Autodesk Inventor part; units mm, degrees
(part 3 of 3)
  spline S597 degree 2 poles (111.3325, 10.8139) (111.3763, 10.2474) (111.3763, 9.9326) knots 0 0 0 1 1 1
  spline S598 degree 2 poles (111.3763, 9.9326) (111.3763, 9.8642) (111.4037, 9.585) (111.4037, 9.5138) knots 0 0 0 1 2 2 2
  spline S599 degree 2 poles (111.4037, 9.5138) (111.4037, 9.3824) (111.3599, 9.2839) knots 0 0 0 1 1 1
  spline S600 degree 2 poles (111.3599, 9.2839) (111.3052, 9.1553) (111.1902, 9.1553) knots 0 0 0 1 1 1
  spline S601 degree 2 poles (111.1902, 9.1553) (111.1108, 9.1553) (110.9849, 9.2648) (110.9849, 9.3523) knots 0 0 0 1 2 2 2
  spline S602 degree 2 poles (110.9849, 9.3523) (110.9849, 9.3824) (111.0041, 9.5001) (111.0041, 9.5275) knots 0 0 0 1 2 2 2
  spline S603 degree 2 poles (111.0041, 9.5275) (111.0041, 9.626) (110.9794, 10.0092) (110.9794, 10.1078) knots 0 0 0 1 2 2 2
  spline S604 degree 2 poles (110.9794, 10.1078) (110.9794, 10.3897) (110.9329, 10.8988) knots 0 0 0 1 1 1
  spline S605 degree 2 poles (110.9329, 10.8988) (110.8864, 11.4462) (110.8809, 11.6871) knots 0 0 0 1 1 1
  line L469 (110.8809, 11.6871) -> (110.703, 11.6843)
  spline S606 degree 2 poles (110.703, 11.6843) (110.2733, 11.6843) (110.0269, 11.7473) knots 0 0 0 1 1 1
  spline S607 degree 2 poles (110.0269, 11.7473) (109.8682, 11.7883) (109.8682, 11.9416) knots 0 0 0 1 1 1
  spline S608 degree 2 poles (109.8682, 11.9416) (109.8682, 12.0237) (109.9202, 12.0839) knots 0 0 0 1 1 1
  spline S609 degree 2 poles (109.9202, 12.0839) (109.9777, 12.1524) (110.0707, 12.1469) knots 0 0 0 1 1 1
  spline S610 degree 2 poles (110.0707, 12.1469) (110.1392, 12.1441) (110.3855, 12.1113) knots 0 0 0 1 1 1
  spline S611 degree 2 poles (110.3855, 12.1113) (110.5798, 12.0867) (110.703, 12.0867) knots 0 0 0 1 1 1
  spline S612 degree 2 poles (110.703, 12.0867) (110.8207, 12.0867) (111.2997, 12.0976) (111.4174, 12.0976) knots 0 0 0 1 2 2 2
  spline S613 degree 2 poles (111.4174, 12.0976) (111.5679, 12.0976) (112.1619, 12.0538) (112.3151, 12.0538) knots 0 0 0 1 2 2 2
  spline S614 degree 2 poles (112.3151, 12.0538) (112.3972, 12.0538) (112.5122, 11.9389) (112.5122, 11.8513) knots 0 0 0 1 2 2 2
  spline S615 degree 2 poles (112.5122, 11.8513) (112.5122, 11.7692) (112.3972, 11.6515) (112.3151, 11.6515) knots 0 0 0 1 2 2 2
  spline S616 degree 2 poles (113.9464, 9.0513) (113.3935, 9.0513) (113.0076, 9.3824) knots 0 0 0 1 1 1
  spline S617 degree 2 poles (113.0076, 9.3824) (112.5998, 9.7355) (112.5998, 10.2939) knots 0 0 0 1 1 1
  spline S618 degree 2 poles (112.5998, 10.2939) (112.5998, 10.9754) (113.0021, 11.531) knots 0 0 0 1 1 1
  spline S619 degree 2 poles (113.0021, 11.531) (113.451, 12.1469) (114.1243, 12.1469) knots 0 0 0 1 1 1
  spline S620 degree 2 poles (114.1243, 12.1469) (114.7675, 12.1469) (115.0823, 11.8568) knots 0 0 0 1 1 1
  spline S621 degree 2 poles (115.0823, 11.8568) (115.4108, 11.5529) (115.4108, 10.9015) knots 0 0 0 1 1 1
  spline S622 degree 2 poles (115.4108, 10.9015) (115.4108, 10.2227) (115.0412, 9.6753) knots 0 0 0 1 1 1
  spline S623 degree 2 poles (115.0412, 9.6753) (114.617, 9.0513) (113.9464, 9.0513) knots 0 0 0 1 1 1
  spline S624 degree 2 poles (114.1243, 11.7445) (113.6426, 11.7445) (113.3087, 11.2655) knots 0 0 0 1 1 1
  spline S625 degree 2 poles (113.3087, 11.2655) (112.9994, 10.8249) (112.9994, 10.2939) knots 0 0 0 1 1 1
  spline S626 degree 2 poles (112.9994, 10.2939) (112.9994, 9.9162) (113.2813, 9.678) knots 0 0 0 1 1 1
  spline S627 degree 2 poles (113.2813, 9.678) (113.5495, 9.4536) (113.9464, 9.4536) knots 0 0 0 1 1 1
  spline S628 degree 2 poles (113.9464, 9.4536) (114.4227, 9.4536) (114.7347, 9.9353) knots 0 0 0 1 1 1
  spline S629 degree 2 poles (114.7347, 9.9353) (115.0111, 10.3651) (115.0111, 10.9015) knots 0 0 0 1 1 1
  spline S630 degree 2 poles (115.0111, 10.9015) (115.0111, 11.3723) (114.8004, 11.5612) knots 0 0 0 1 1 1
  spline S631 degree 2 poles (114.8004, 11.5612) (114.6006, 11.7445) (114.1243, 11.7445) knots 0 0 0 1 1 1
  spline S632 degree 2 poles (102.0155, 2.4094) (101.9416, 2.4094) (101.8759, 2.4724) knots 0 0 0 1 1 1
  spline S633 degree 2 poles (101.8759, 2.4724) (101.2273, 3.1128) (100.4308, 3.3345) knots 0 0 0 1 1 1
  line L470 (100.4308, 3.3345) -> (100.4472, 2.9513)
  line L471 (100.4472, 2.9513) -> (100.4581, 2.5654)
  spline S634 degree 2 poles (100.4581, 2.5654) (100.4581, 2.4778) (100.3459, 2.3629) (100.2611, 2.3629) knots 0 0 0 1 2 2 2
  spline S635 degree 2 poles (100.2611, 2.3629) (100.1762, 2.3629) (100.064, 2.4778) (100.064, 2.5654) knots 0 0 0 1 2 2 2
  spline S636 degree 2 poles (100.064, 2.5654) (100.064, 2.7214) (100.0339, 3.3345) (100.0339, 3.4905) knots 0 0 0 1 2 2 2
  spline S637 degree 2 poles (100.0339, 3.4905) (100.0339, 3.6712) (100.1133, 4.3856) (100.1133, 4.5635) knots 0 0 0 1 2 2 2
  spline S638 degree 2 poles (100.1133, 4.5635) (100.1133, 4.6647) (100.075, 5.0561) (100.075, 5.1574) knots 0 0 0 1 2 2 2
  spline S639 degree 2 poles (100.075, 5.1574) (100.075, 5.2696) (100.1379, 5.3545) knots 0 0 0 1 1 1
  spline S640 degree 2 poles (100.1379, 5.3545) (100.2118, 5.4585) (100.3432, 5.4475) knots 0 0 0 1 1 1
  line L472 (100.3432, 5.4475) -> (100.8167, 5.4092)
  spline S641 degree 2 poles (100.8167, 5.4092) (101.0849, 5.3764) (101.2711, 5.2778) knots 0 0 0 1 1 1
  spline S642 degree 2 poles (101.2711, 5.2778) (102.0648, 4.8563) (102.0648, 4.2487) knots 0 0 0 1 1 1
  spline S643 degree 2 poles (102.0648, 4.2487) (102.0648, 3.9504) (101.7938, 3.7205) knots 0 0 0 1 1 1
  spline S644 degree 2 poles (101.7938, 3.7205) (101.5776, 3.5343) (101.2519, 3.4385) knots 0 0 0 1 1 1
  spline S645 degree 2 poles (101.2519, 3.4385) (101.8623, 3.1101) (102.1633, 2.7461) knots 0 0 0 1 1 1
  spline S646 degree 2 poles (102.1633, 2.7461) (102.2153, 2.6831) (102.2153, 2.6147) knots 0 0 0 1 1 1
  spline S647 degree 2 poles (102.2153, 2.6147) (102.2153, 2.5298) (102.0949, 2.4094) (102.0155, 2.4094) knots 0 0 0 1 2 2 2
  line L473 (100.7647, 5.0041) -> (100.4746, 5.0288)
  line L474 (100.4746, 5.0288) -> (100.4937, 4.7907)
  spline S648 degree 2 poles (100.4937, 4.7907) (100.5074, 4.6456) (100.5074, 4.5525) knots 0 0 0 1 1 1
  spline S649 degree 2 poles (100.5074, 4.5525) (100.5074, 4.3965) (100.4828, 4.1611) knots 0 0 0 1 1 1
  line L475 (100.4828, 4.1611) -> (100.4417, 3.7697)
  spline S650 degree 2 poles (100.4417, 3.7697) (100.4691, 3.7697) (100.5841, 3.767) (100.6142, 3.767) knots 0 0 0 1 2 2 2
  spline S651 degree 2 poles (100.6142, 3.767) (101.115, 3.767) (101.3641, 3.9011) knots 0 0 0 1 1 1
  spline S652 degree 2 poles (101.3641, 3.9011) (101.4736, 3.9613) (101.5667, 4.0599) knots 0 0 0 1 1 1
  spline S653 degree 2 poles (101.5667, 4.0599) (101.6707, 4.1693) (101.6707, 4.246) knots 0 0 0 1 1 1
  spline S654 degree 2 poles (101.6707, 4.246) (101.6707, 4.5197) (101.3614, 4.7551) knots 0 0 0 1 1 1
  spline S655 degree 2 poles (101.3614, 4.7551) (101.0767, 4.9713) (100.7647, 5.0041) knots 0 0 0 1 1 1
  spline S656 degree 2 poles (103.9041, 2.3109) (103.3512, 2.3109) (102.9653, 2.6421) knots 0 0 0 1 1 1
  spline S657 degree 2 poles (102.9653, 2.6421) (102.5575, 2.9951) (102.5575, 3.5535) knots 0 0 0 1 1 1
  spline S658 degree 2 poles (102.5575, 3.5535) (102.5575, 4.235) (102.9598, 4.7907) knots 0 0 0 1 1 1
  spline S659 degree 2 poles (102.9598, 4.7907) (103.4087, 5.4065) (104.082, 5.4065) knots 0 0 0 1 1 1
  spline S660 degree 2 poles (104.082, 5.4065) (104.7252, 5.4065) (105.04, 5.1164) knots 0 0 0 1 1 1
  spline S661 degree 2 poles (105.04, 5.1164) (105.3684, 4.8125) (105.3684, 4.1611) knots 0 0 0 1 1 1
  spline S662 degree 2 poles (105.3684, 4.1611) (105.3684, 3.4823) (104.9989, 2.9349) knots 0 0 0 1 1 1
  spline S663 degree 2 poles (104.9989, 2.9349) (104.5747, 2.3109) (103.9041, 2.3109) knots 0 0 0 1 1 1
  spline S664 degree 2 poles (104.082, 5.0041) (103.6003, 5.0041) (103.2664, 4.5252) knots 0 0 0 1 1 1
  spline S665 degree 2 poles (103.2664, 4.5252) (102.9571, 4.0845) (102.9571, 3.5535) knots 0 0 0 1 1 1
  spline S666 degree 2 poles (102.9571, 3.5535) (102.9571, 3.1758) (103.239, 2.9377) knots 0 0 0 1 1 1
  spline S667 degree 2 poles (103.239, 2.9377) (103.5072, 2.7132) (103.9041, 2.7132) knots 0 0 0 1 1 1
  spline S668 degree 2 poles (103.9041, 2.7132) (104.3804, 2.7132) (104.6924, 3.1949) knots 0 0 0 1 1 1
  spline S669 degree 2 poles (104.6924, 3.1949) (104.9688, 3.6247) (104.9688, 4.1611) knots 0 0 0 1 1 1
  spline S670 degree 2 poles (104.9688, 4.1611) (104.9688, 4.6319) (104.7581, 4.8208) knots 0 0 0 1 1 1
  spline S671 degree 2 poles (104.7581, 4.8208) (104.5583, 5.0041) (104.082, 5.0041) knots 0 0 0 1 1 1
  spline S672 degree 2 poles (107.2789, 2.5107) (106.8383, 2.3382) (106.1512, 2.3382) knots 0 0 0 1 1 1
  spline S673 degree 2 poles (106.1512, 2.3382) (106.0664, 2.3382) (105.9159, 2.497) (105.9159, 2.5818) knots 0 0 0 1 2 2 2
  line L476 (105.9159, 2.5818) -> (105.9159, 3.1539)
  spline S674 degree 2 poles (105.9159, 3.1539) (105.9159, 3.4331) (105.9514, 3.9531) knots 0 0 0 1 1 1
  spline S675 degree 2 poles (105.9514, 3.9531) (105.9898, 4.5142) (105.9925, 4.766) knots 0 0 0 1 1 1
  spline S676 degree 2 poles (105.9925, 4.766) (105.9925, 4.9467) (106.0144, 5.3052) knots 0 0 0 1 1 1
  spline S677 degree 2 poles (106.0144, 5.3052) (106.0281, 5.401) (106.0801, 5.4339) knots 0 0 0 1 1 1
  spline S678 degree 2 poles (106.0801, 5.4339) (106.3456, 5.516) (106.685, 5.516) knots 0 0 0 1 1 1
  spline S679 degree 2 poles (106.685, 5.516) (107.0326, 5.516) (107.3501, 5.2806) knots 0 0 0 1 1 1
  spline S680 degree 2 poles (107.3501, 5.2806) (107.7169, 5.0096) (107.7169, 4.61) knots 0 0 0 1 1 1
  spline S681 degree 2 poles (107.7169, 4.61) (107.7169, 4.1064) (107.3255, 3.8163) knots 0 0 0 1 1 1
  spline S682 degree 2 poles (107.3255, 3.8163) (107.6183, 3.6903) (107.9112, 3.3838) (107.9112, 3.2032) knots 0 0 0 1 2 2 2
  spline S683 degree 2 poles (107.9112, 3.2032) (107.9112, 2.965) (107.6539, 2.7433) knots 0 0 0 1 1 1
  spline S684 degree 2 poles (107.6539, 2.7433) (107.476, 2.5873) (107.2789, 2.5107) knots 0 0 0 1 1 1
  spline S685 degree 2 poles (106.6877, 5.1164) (106.4742, 5.1164) (106.3866, 5.1027) knots 0 0 0 1 1 1
  line L477 (106.3866, 5.1027) -> (106.3839, 4.7578)
  line L478 (106.3839, 4.7578) -> (106.3428, 3.9969)
  spline S686 degree 2 poles (106.3428, 3.9969) (106.622, 3.9723) (106.6412, 3.975) knots 0 0 0 1 1 1
  spline S687 degree 2 poles (106.6412, 3.975) (106.9368, 3.9996) (107.1256, 4.1611) knots 0 0 0 1 1 1
  spline S688 degree 2 poles (107.1256, 4.1611) (107.3282, 4.3363) (107.3282, 4.61) knots 0 0 0 1 1 1
  spline S689 degree 2 poles (107.3282, 4.61) (107.3282, 4.7989) (106.9176, 5.1164) (106.6877, 5.1164) knots 0 0 0 1 2 2 2
  line L479 (106.9067, 3.5425) -> (106.6987, 3.5754)
  spline S690 degree 2 poles (106.6987, 3.5754) (106.674, 3.5754) (106.57, 3.5699) (106.5427, 3.5699) knots 0 0 0 1 2 2 2
  spline S691 degree 2 poles (106.5427, 3.5699) (106.4359, 3.5699) (106.3155, 3.5863) knots 0 0 0 1 1 1
  spline S692 degree 2 poles (106.3155, 3.5863) (106.3045, 3.34) (106.3045, 3.1457) knots 0 0 0 1 1 1
  line L480 (106.3045, 3.1457) -> (106.3045, 2.7406)
  spline S693 degree 2 poles (106.3045, 2.7406) (106.8191, 2.757) (107.1421, 2.8857) knots 0 0 0 1 1 1
  spline S694 degree 2 poles (107.1421, 2.8857) (107.2789, 2.9377) (107.4048, 3.0499) knots 0 0 0 1 1 1
  spline S695 degree 2 poles (107.4048, 3.0499) (107.5253, 3.1511) (107.5253, 3.2032) knots 0 0 0 1 1 1
  spline S696 degree 2 poles (107.5253, 3.2032) (107.5253, 3.2962) (107.2734, 3.4112) knots 0 0 0 1 1 1
  spline S697 degree 2 poles (107.2734, 3.4112) (107.0846, 3.4988) (106.9067, 3.5425) knots 0 0 0 1 1 1
  spline S698 degree 2 poles (109.6492, 2.3109) (109.0963, 2.3109) (108.7104, 2.6421) knots 0 0 0 1 1 1
  spline S699 degree 2 poles (108.7104, 2.6421) (108.3026, 2.9951) (108.3026, 3.5535) knots 0 0 0 1 1 1
  spline S700 degree 2 poles (108.3026, 3.5535) (108.3026, 4.235) (108.7049, 4.7907) knots 0 0 0 1 1 1
  spline S701 degree 2 poles (108.7049, 4.7907) (109.1538, 5.4065) (109.8271, 5.4065) knots 0 0 0 1 1 1
  spline S702 degree 2 poles (109.8271, 5.4065) (110.4703, 5.4065) (110.7851, 5.1164) knots 0 0 0 1 1 1
  spline S703 degree 2 poles (110.7851, 5.1164) (111.1136, 4.8125) (111.1136, 4.1611) knots 0 0 0 1 1 1
  spline S704 degree 2 poles (111.1136, 4.1611) (111.1136, 3.4823) (110.7441, 2.9349) knots 0 0 0 1 1 1
  spline S705 degree 2 poles (110.7441, 2.9349) (110.3198, 2.3109) (109.6492, 2.3109) knots 0 0 0 1 1 1
  spline S706 degree 2 poles (109.8271, 5.0041) (109.3454, 5.0041) (109.0115, 4.5252) knots 0 0 0 1 1 1
  spline S707 degree 2 poles (109.0115, 4.5252) (108.7022, 4.0845) (108.7022, 3.5535) knots 0 0 0 1 1 1
  spline S708 degree 2 poles (108.7022, 3.5535) (108.7022, 3.1758) (108.9841, 2.9377) knots 0 0 0 1 1 1
  spline S709 degree 2 poles (108.9841, 2.9377) (109.2523, 2.7132) (109.6492, 2.7132) knots 0 0 0 1 1 1
  spline S710 degree 2 poles (109.6492, 2.7132) (110.1255, 2.7132) (110.4375, 3.1949) knots 0 0 0 1 1 1
  spline S711 degree 2 poles (110.4375, 3.1949) (110.7139, 3.6247) (110.7139, 4.1611) knots 0 0 0 1 1 1
  spline S712 degree 2 poles (110.7139, 4.1611) (110.7139, 4.6319) (110.5032, 4.8208) knots 0 0 0 1 1 1
  spline S713 degree 2 poles (110.5032, 4.8208) (110.3034, 5.0041) (109.8271, 5.0041) knots 0 0 0 1 1 1
  spline S714 degree 2 poles (113.9601, 4.9111) (113.815, 4.9111) (113.5112, 4.9357) knots 0 0 0 1 1 1
  spline S715 degree 2 poles (113.5112, 4.9357) (113.2184, 4.9576) (113.0651, 4.9549) knots 0 0 0 1 1 1
  line L481 (113.0651, 4.9549) -> (112.9255, 4.9549)
  spline S716 degree 2 poles (112.9255, 4.9549) (112.931, 4.6839) (112.9775, 4.0735) knots 0 0 0 1 1 1
  spline S717 degree 2 poles (112.9775, 4.0735) (113.0213, 3.507) (113.0213, 3.1922) knots 0 0 0 1 1 1
  spline S718 degree 2 poles (113.0213, 3.1922) (113.0213, 3.1238) (113.0487, 2.8446) (113.0487, 2.7734) knots 0 0 0 1 2 2 2
  spline S719 degree 2 poles (113.0487, 2.7734) (113.0487, 2.6421) (113.0049, 2.5435) knots 0 0 0 1 1 1
  spline S720 degree 2 poles (113.0049, 2.5435) (112.9501, 2.4149) (112.8352, 2.4149) knots 0 0 0 1 1 1
  spline S721 degree 2 poles (112.8352, 2.4149) (112.7558, 2.4149) (112.6299, 2.5244) (112.6299, 2.6119) knots 0 0 0 1 2 2 2
  spline S722 degree 2 poles (112.6299, 2.6119) (112.6299, 2.6421) (112.6491, 2.7597) (112.6491, 2.7871) knots 0 0 0 1 2 2 2
  spline S723 degree 2 poles (112.6491, 2.7871) (112.6491, 2.8857) (112.6244, 3.2688) (112.6244, 3.3674) knots 0 0 0 1 2 2 2
  spline S724 degree 2 poles (112.6244, 3.3674) (112.6244, 3.6493) (112.5779, 4.1584) knots 0 0 0 1 1 1
  spline S725 degree 2 poles (112.5779, 4.1584) (112.5314, 4.7058) (112.5259, 4.9467) knots 0 0 0 1 1 1
  line L482 (112.5259, 4.9467) -> (112.348, 4.9439)
  spline S726 degree 2 poles (112.348, 4.9439) (111.9183, 4.9439) (111.6719, 5.0069) knots 0 0 0 1 1 1
  spline S727 degree 2 poles (111.6719, 5.0069) (111.5132, 5.0479) (111.5132, 5.2012) knots 0 0 0 1 1 1
  spline S728 degree 2 poles (111.5132, 5.2012) (111.5132, 5.2833) (111.5652, 5.3435) knots 0 0 0 1 1 1
  spline S729 degree 2 poles (111.5652, 5.3435) (111.6227, 5.412) (111.7157, 5.4065) knots 0 0 0 1 1 1
  spline S730 degree 2 poles (111.7157, 5.4065) (111.7841, 5.4038) (112.0305, 5.3709) knots 0 0 0 1 1 1
  spline S731 degree 2 poles (112.0305, 5.3709) (112.2248, 5.3463) (112.348, 5.3463) knots 0 0 0 1 1 1
  spline S732 degree 2 poles (112.348, 5.3463) (112.4657, 5.3463) (112.9447, 5.3572) (113.0623, 5.3572) knots 0 0 0 1 2 2 2
  spline S733 degree 2 poles (113.0623, 5.3572) (113.2129, 5.3572) (113.8068, 5.3134) (113.9601, 5.3134) knots 0 0 0 1 2 2 2
  spline S734 degree 2 poles (113.9601, 5.3134) (114.0422, 5.3134) (114.1572, 5.1985) (114.1572, 5.1109) knots 0 0 0 1 2 2 2
  spline S735 degree 2 poles (114.1572, 5.1109) (114.1572, 5.0288) (114.0422, 4.9111) (113.9601, 4.9111) knots 0 0 0 1 2 2 2
  spline S736 degree 2 poles (115.5914, 2.3109) (115.0385, 2.3109) (114.6526, 2.6421) knots 0 0 0 1 1 1
  spline S737 degree 2 poles (114.6526, 2.6421) (114.2448, 2.9951) (114.2448, 3.5535) knots 0 0 0 1 1 1
  spline S738 degree 2 poles (114.2448, 3.5535) (114.2448, 4.235) (114.6471, 4.7907) knots 0 0 0 1 1 1
  spline S739 degree 2 poles (114.6471, 4.7907) (115.096, 5.4065) (115.7693, 5.4065) knots 0 0 0 1 1 1
  spline S740 degree 2 poles (115.7693, 5.4065) (116.4125, 5.4065) (116.7273, 5.1164) knots 0 0 0 1 1 1
  spline S741 degree 2 poles (116.7273, 5.1164) (117.0557, 4.8125) (117.0557, 4.1611) knots 0 0 0 1 1 1
  spline S742 degree 2 poles (117.0557, 4.1611) (117.0557, 3.4823) (116.6862, 2.9349) knots 0 0 0 1 1 1
  spline S743 degree 2 poles (116.6862, 2.9349) (116.262, 2.3109) (115.5914, 2.3109) knots 0 0 0 1 1 1
  spline S744 degree 2 poles (115.7693, 5.0041) (115.2876, 5.0041) (114.9537, 4.5252) knots 0 0 0 1 1 1
  spline S745 degree 2 poles (114.9537, 4.5252) (114.6444, 4.0845) (114.6444, 3.5535) knots 0 0 0 1 1 1
  spline S746 degree 2 poles (114.6444, 3.5535) (114.6444, 3.1758) (114.9263, 2.9377) knots 0 0 0 1 1 1
  spline S747 degree 2 poles (114.9263, 2.9377) (115.1945, 2.7132) (115.5914, 2.7132) knots 0 0 0 1 1 1
  spline S748 degree 2 poles (115.5914, 2.7132) (116.0677, 2.7132) (116.3797, 3.1949) knots 0 0 0 1 1 1
  spline S749 degree 2 poles (116.3797, 3.1949) (116.6561, 3.6247) (116.6561, 4.1611) knots 0 0 0 1 1 1
  spline S750 degree 2 poles (116.6561, 4.1611) (116.6561, 4.6319) (116.4454, 4.8208) knots 0 0 0 1 1 1
  spline S751 degree 2 poles (116.4454, 4.8208) (116.2456, 5.0041) (115.7693, 5.0041) knots 0 0 0 1 1 1
  point P0 (-0.7071, -3)
  dimension "PitchL" = 41.0031
  dimension "PitchW" = 34.3586
  dimension "NWellsL" = 3
  dimension "NWellsW" = 2
  dimension "OffsetL" = 2.75
  dimension "OffsetW" = 6
  dimension "WallThickL" = 1.75
  dimension "WallThickW" = 5
  dimension "WellRadius" = 7.4295
  constraints: 4 other
emboss "Emboss2" sketch "Sketch5" operation cut depth 1 direction (-1, 0, 0)
equation "\"d6\" = RimOffset"
equation "\"d51\" = WallThickW"
equation "\"d63\" = WallThickL"
equation "\"d64\" = BlockW"
equation "\"d65\" = BlockL"
equation "\"WellDepth\" = WellSectionH"
equation "\"d58\" = PitchW"
equation "\"d61\" = PitchL"
equation "\"PitchL\" = BlockL + 2 * WallThickL"
equation "\"PitchW\" = BlockW + 2 * WallThickW"
equation "\"OffsetL\" = RimOffset + WallThickL"
equation "\"OffsetW\" = RimOffset + WallThickW"
equation "\"WallThickL\" = 1.75"
equation "\"WallThickW\" = 5"
equation "\"WellRadius\" = 0.5 * WellDiameter"
equation "\"WellDiameter\" = 14.859"
equation "\"BlockL\" = TrueBlockL + BlockFitTolerance"
equation "\"BlockW\" = TrueBlockW + BlockFitTolerance"
equation "\"TrueBlockL\" = 34.9631"
equation "\"TrueBlockW\" = 21.8186"
equation "\"BlockFitTolerance\" = 2.54"
equation "\"WellSectionH\" = 30"
body "Solid1"
